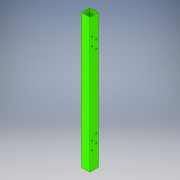
# Autodesk Inventor part: ElvEndEffectBeam
Saved by Autodesk Inventor 2019 (Build 230136000, 136)
## iProperties
Created: 2019-01-09
Part Number: ElvEndEffectBeam
Material: Aluminum 6061
Document SubType Name: Modeling
Designer: james
Density: 2.7 g/cm^3
Appearance: Default(2)
Mass: 134.652 g
Surface Area: 631.805 cm^2
Volume: 49.8713 cm^3
Author: james
Autodesk Inventor part; units mm, degrees
ref_plane "YZ Plane" through (0, 0, 0) normal (1, 0, 0) x (0, 1, 0)
ref_plane "XZ Plane" through (0, 0, 0) normal (0, 1, 0) x (-1, 0, 0)
ref_plane "XY Plane" through (0, 0, 0) normal (0, 0, 1) x (1, 0, 0)
sketch "Sketch1" plane through (0, 0, 0) normal (0, 1, 0) x (-1, 0, 0)
  line L0 (17.0295, 14.999) -> (-8.3705, 14.999)
  line L1 (-8.3705, 14.999) -> (-8.3705, -10.401)
  line L2 (-8.3705, -10.401) -> (17.0295, -10.401)
  line L3 (17.0295, -10.401) -> (17.0295, 14.999)
  line L4 (15.442, -8.8135) -> (-6.783, -8.8135)
  line L5 (-6.783, -8.8135) -> (-6.783, 13.4115)
  line L6 (-6.783, 13.4115) -> (15.442, 13.4115)
  line L7 (15.442, 13.4115) -> (15.442, -8.8135)
  point P0 (0, 0)
  dimension "d0" = 25.4
  dimension "d1" = 25.4
  dimension "d4" = 1.5875
  dimension "d5" = 1.5875
  dimension "d6" = 1.5875
  dimension "d7" = 1.5875
  constraints: 16 end point, 4 parallel, 2 horizontal, 2 perpendicular
  measures "d0" distance of L0.end L1.end
  measures "d1" distance of L0.start L0.end
  measures "d4" distance between parallel lines of L0 L6
  measures "d5" distance between parallel lines of L2 L4
  measures "d6" distance between parallel lines of L3 L7
  measures "d7" distance between parallel lines of L1 L5
extrude "Extrusion2" add sketch "Sketch1" along normal blind 406.4
sketch "Sketch3" plane through (8.3705, 0, 14.999) normal (1, 0, 0) x (0, 0, -1)
  line L0 (25.4, 0) -> (25.4, 406.4) projected
  line L1 (0, 406.4) -> (25.4, 406.4) projected
  line L2 (0, 0) -> (25.4, 0) projected
  point P0 (14.999, 0)
  point P1 (19.05, 339.725)
  point P2 (19.05, 66.675)
  dimension "d19" = 6.35
  dimension "d20" = 66.675
  dimension "d21" = 6.35
  dimension "d22" = 66.675
  measures "d19" distance from line of L0 point (19.05, 339.725)
  measures "d20" distance from line of L1 point (19.05, 339.725)
  measures "d21" distance from line of L0 point (19.05, 66.675)
  measures "d22" distance from line of L2 point (19.05, 66.675)
hole "Hole2" at (8.3705, 339.725, -4.051) at (8.3705, 66.675, -4.051) direction (-1, 0, 0) diameter 4.7625 depth 25.4 tip angle 118.188
sketch "Sketch4" plane through (8.3705, 0, 14.999) normal (1, 0, 0) x (0, 0, -1)
  line L0 (25.4, 0) -> (25.4, 406.4) projected
  circle A0 centre (19.05, 66.675) radius 2.3813 projected
  line L1 (0, 0) -> (0, 406.4) projected
  circle A1 centre (19.05, 339.725) radius 2.3813 projected
  point P0 (14.999, 0)
  point P1 (19.05, 92.075)
  point P2 (6.35, 53.975)
  point P3 (6.35, 79.375)
  point P4 (19.05, 314.325)
  point P5 (6.35, 352.425)
  point P6 (6.35, 327.025)
  dimension "d30" = 6.35
  dimension "d31" = 25.4
  dimension "d32" = 6.35
  dimension "d33" = 6.35
  dimension "d34" = 25.4
  dimension "d36" = 6.35
  dimension "d37" = 25.4
  dimension "d38" = 6.35
  dimension "d39" = 6.35
  dimension "d40" = 25.4
  dimension "d49" = 12.7
  dimension "d50" = 12.7
  measures "d30" distance from line of L0 point (19.05, 92.075)
  measures "d31" distance of A0.centre point (19.05, 92.075)
  measures "d32" distance from line of L1 point (6.35, 79.375)
  measures "d33" distance from line of L1 point (6.35, 53.975)
  measures "d34" distance of point (6.35, 79.375) point (6.35, 53.975)
  measures "d36" distance from line of L0 point (19.05, 314.325)
  measures "d37" distance of A1.centre point (19.05, 314.325)
  measures "d38" distance from line of L1 point (6.35, 352.425)
  measures "d39" distance from line of L1 point (6.35, 327.025)
  measures "d40" distance of point (6.35, 352.425) point (6.35, 327.025)
  measures "d49" horizontal distance of point (6.35, 327.025) point (19.05, 314.325)
  measures "d50" horizontal distance of point (6.35, 53.975) A0.centre
hole "Hole3" at (8.3705, 92.075, -4.051) at (8.3705, 53.975, 8.649) at (8.3705, 79.375, 8.649) at (8.3705, 314.325, -4.051) at (8.3705, 352.425, 8.649) at (8.3705, 327.025, 8.649) direction (-1, 0, 0) diameter 4.7625 depth 25.4 tip angle 118.188
equation "\"d0\" = ElvBeamWidth"
equation "\"d1\" = ElvBeamWidth"
equation "\"d4\" = ElvWallWidth"
equation "\"d5\" = ElvWallWidth"
equation "\"d6\" = ElvWallWidth"
equation "\"d7\" = ElvWallWidth"
equation "\"d8\" = ElvEndEffectLength"
equation "\"ElvMiddleBeamLength\" = 990.6"
equation "\"ElvWallWidth\" = 1.5875"
equation "\"ElvFrontBeamLength\" = 990.6"
equation "\"ElvEndEffectLength\" = 406.4"
equation "\"ElvCrossBeamLength\" = 304.8"
equation "\"ElvBeamWidth\" = 25.4"
equation "\"ElvFrontBeamLength_1\" = 1066.8"
equation "\"ElvFixedBeamLength\" = 990.6"
equation "\"ElvDelHeight\" = 101.6"
equation "\"ElvDelFrontTabLength\" = 6.35"
equation "\"ElvDelWidth\" = 18.542"
equation "\"ElvDelDepth\" = 6.35"
equation "\"ElvTopBeamLength\" = 457.2"
equation "\"ElvHoleFromFixed\" = 50.8"
equation "\"ElvHoleFromMid\" = 38.1"
equation "\"ElvHoleFromFront\" = 25.4"
equation "\"ElvHoleFromBottom\" = 38.1"
equation "\"ElvRivetPlateLength\" = 76.2"
equation "\"ElvDelMiddleTabLength\" = 6.35"
body "Solid2"
